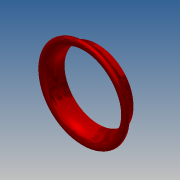
# Autodesk Inventor part: A1-19027-500-02 HCWI nozzle horn
Saved by Autodesk Inventor 2017.3 (Build 213257000, 257)
## iProperties
Created: 2018-10-30
Part Number: A1-19027-500-02 HCWI nozzle horn
Material: Iron, HCWI
Document SubType Name: Modeling
Designer: Graeme_Van_Dongen
Density: 7.33517 g/cm^3
Appearance: Iron Gray(1)
Mass: 146650 g
Surface Area: 12477.7 cm^2
Volume: 19992.8 cm^3
Description: Ø28 1/2" ID x 1 3/16" WALL x 7 3/32" FLARE TO Ø37 25/32" OD HCWI HORN, ASTM A532 CLASS III TYPE A, PF# 470294
Author: Graeme_Van_Dongen
Autodesk Inventor part; units mm, degrees
ref_plane "YZ Plane" through (0, 0, 0) normal (1, 0, 0) x (0, 1, 0)
ref_plane "XZ Plane" through (0, 0, 0) normal (0, 1, 0) x (-1, 0, 0)
ref_plane "XY Plane" through (0, 0, 0) normal (0, 0, 1) x (1, 0, 0)
sketch "Sketch1" plane through (0, 0, 0) normal (0, 0, 1) x (1, 0, 0)
  line L0 (0, 0) -> (19.0759, 0)
  line L1 (19.0759, 390.525) -> (0, 390.525)
  line L2 (0, 390.525) -> (0, 361.95)
  line L3 (0, 361.95) -> (19.0759, 361.95)
  line L4 (19.0759, 361.95) -> (19.0759, 390.525)
  arc A0 (-62.453, 370.1721) -> (0, 361.95) centre (0, 603.25) ccw
  arc A1 (-109.1582, 392.2246) -> (-62.453, 370.1721) centre (-24.9812, 510.0188) ccw
  arc A2 (-136.5303, 424.4172) -> (-109.1582, 392.2246) centre (-58.652, 462.9011) ccw
  arc A3 (-141.6085, 453.2354) -> (-136.5303, 424.4172) centre (-89.8033, 447.5076) ccw
  line L5 (0, 603.25) -> (-62.453, 370.1721) construction
  line L6 (-24.9812, 510.0188) -> (-109.1582, 392.2246) construction
  line L7 (-58.652, 462.9011) -> (-136.5303, 424.4172) construction
  line L8 (-97.5912, 443.6592) -> (-141.6085, 453.2354) construction
  arc A4 (-123.6848, 478.1677) -> (-141.6085, 453.2354) centre (-110.5254, 449.7987) ccw
  line L9 (-110.5254, 449.7987) -> (-123.6848, 478.1677) construction
  line L10 (-141.9241, 481.0712) -> (-141.9241, 0) construction
  arc A5 (-97.3107, 464.4045) -> (-123.6848, 478.1677) centre (-115.7891, 461.1463) ccw
  line L11 (-115.7891, 461.1463) -> (-97.3107, 464.4045) construction
  arc A6 (-97.3107, 464.4045) -> (-82.4862, 430.9434) centre (-22.2684, 477.6365) ccw
  arc A7 (-82.4862, 430.9434) -> (0, 390.525) centre (0, 494.9035) ccw
  line L12 (-110.5254, 449.7987) -> (-110.5254, 481.0712) construction
  dimension "d1" = 781.05
  dimension "d3" = 723.9
  dimension "d4" = 723.9
  dimension "d5" = 241.3
  dimension "d6" = 15
  dimension "d7" = 144.78
  dimension "d8" = 20.55
  dimension "d9" = 86.868
  dimension "d10" = 28.154
  dimension "d11" = 52.1208
  dimension "d12" = 38.57
  dimension "d13" = 31.2725
  dimension "d14" = 52.841
  dimension "d17" = 18.7635
  dimension "d18" = 80
  dimension "d19" = 76.2
  dimension "d37" = 0
  dimension "d94" = 962.1424
  dimension "d99" = 161
  dimension "d100" = 19.0758
  dimension "d101" = 895.0151
  dimension "d112" = 19.0758
  constraints: 26 end point, 17 point on circle, 10 tangent, 8 centre point, 2 horizontal, 2 horizontal alignment, 2 perpendicular, 2 point on line, 2 vertical, 1 midpoint
  measures "d1" diameter of L1 L0
  measures "d3" diameter of L3.end L0
  measures "d4" diameter of L2.end L0
  measures "d5" radius of A0
  measures "d6" angle of L2 L5
  measures "d7" radius of A1
  measures "d8" angle of L5 L6
  measures "d9" radius of A2
  measures "d10" angle of L6 L7
  measures "d11" radius of A3
  measures "d12" angle of L7 L8
  measures "d13" radius of A4
  measures "d14" angle of L8 L9
  measures "d17" radius of A5
  measures "d18" angle of L2 L11
  measures "d19" radius of A6
  measures "d37" angle of L1 L3
  measures "d94" diameter of L12.end L0
  measures "d100" distance of L0.start L0.end
  measures "d101" diameter of A3.centre L0
  measures "d112" distance of L1.start L1.end
revolve "Revolution1" add sketch "Sketch1" angle 360 about axis through (0, 0, 0) along (1, 0, 0)
sketch "Sketch9" plane through (19.0759, 0, 0) normal (1, 0, 0) x (0, 0, -1)
  circle A0 centre (0, 0) radius 390.525 projected
  circle A1 centre (0, 0) radius 387.5532
  circle A2 centre (0, 0) radius 430.9434 projected
  dimension "d95" = 775.1064
  constraints: 1 centre point, 1 coincident
  measures "d95" diameter of A1
extrude "Extrusion8" cut sketch "Sketch9" against normal blind 34.925 contours A0 | A2
fillet "Fillet14" radius 0.7937 1 edges at (-15.8491, 0, 387.5532)
sketch "Sketch11" plane through (19.0759, 0, 0) normal (1, 0, 0) x (0, 0, -1)
  circle A0 centre (0, 0) radius 361.95 projected
  circle A1 centre (0, 0) radius 387.5532 projected
extrude "Extrusion10" add sketch "Sketch11" along normal blind 6.35
sketch "Sketch10" plane through (25.4259, 0, 0) normal (1, 0, 0) x (0, 0, -1)
  circle A0 centre (0, 0) radius 374.396
  circle A1 centre (0, 0) radius 361.95 projected
  dimension "d111" = 12.446
  constraints: 1 centre point, 1 coincident
  measures "d111" radial gap between concentric circles of A1 A0
extrude "Extrusion9" add sketch "Sketch10" along normal blind 12.7
fillet "Fillet15" radius 0.7937 1 edges at (25.4259, 0, 374.396)
chamfer "Chamfer4" distance 0.7937 angle 45 1 edges at (38.1259, 0, 374.396)
equation "\"Curve_Ratio\" = 0.6"
equation "\"Angle_Ratio\" = 1.37"
body "Solid1"
